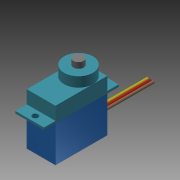
# Autodesk Inventor part: servo-micro tower pro 9g
Saved by Autodesk Inventor 2015 SP2 (Build 190223200, 223)
## iProperties
Created: 2015-05-24
Part Number: servo-micro tower pro 9g
Material: Generic
Document SubType Name: Modeling
Designer: caleb
Density: 1 g/cm^3
Appearance: Default
Author: caleb
Autodesk Inventor part; units mm, degrees
ref_plane "YZ Plane" through (0, 0, 0) normal (1, 0, 0) x (0, 1, 0)
ref_plane "XZ Plane" through (0, 0, 0) normal (0, 1, 0) x (-1, 0, 0)
ref_plane "XY Plane" through (0, 0, 0) normal (0, 0, 1) x (1, 0, 0)
sketch "Sketch1" plane through (0, 0, 0) normal (0, 0, 1) x (1, 0, 0)
  line L0 (-6.35, -16.51) -> (6.35, -16.51)
  line L1 (6.35, -16.51) -> (6.35, 0)
  line L2 (6.35, 6.35) -> (-6.35, 6.35)
  line L3 (-6.35, 6.35) -> (-6.35, 0)
  circle A0 centre (0, 0) radius 6.35
  line L4 (-6.35, 0) -> (-6.35, -16.51)
  line L5 (6.35, 0) -> (6.35, 6.35)
  circle A1 centre (0, 0) radius 2.286
  point P0 (0, 6.35)
  dimension "d0" = 12.7
  dimension "d1" = 22.86
  dimension "d3" = 4.572
  constraints: 12 end point, 5 parallel, 3 tangent, 2 centre point, 2 coincident, 2 perpendicular, 2 point on circle, 1 horizontal, 1 midpoint, 1 vertical alignment
  measures "d0" distance of L0.start L0.end
  measures "d1" distance of L0.end L2.start
  measures "d3" diameter of A1
extrude "Extrusion1" add sketch "Sketch1" against normal blind 16.002 contours L4 A0 L1 L0 | A0 | L3 L2 A0 | A0 L2 L5 | A1
extrude "Extrusion2" add sketch "Sketch1" along normal blind 6.731 separate body contours L4 A0 L1 L0 | A0 | L3 L2 A0 | A0 L2 L5 | A1
sketch "Sketch2" plane through (0, 0, 6.731) normal (0, 0, 1) x (1, 0, 0)
  circle A0 centre (0, 0) radius 6.35 projected
  circle A1 centre (0, 0) radius 2.286 projected
sketch "Sketch3" plane through (0, 0, 0) normal (0, 0, 1) x (1, 0, 0)
  line L0 (-6.35, 6.35) -> (6.35, 6.35)
  line L1 (6.35, 6.35) -> (6.35, 11.43)
  line L2 (6.35, 11.43) -> (-6.35, 11.43)
  line L3 (-6.35, 11.43) -> (-6.35, 6.35)
  line L4 (-6.35, -16.51) -> (6.35, -16.51)
  line L5 (6.35, -16.51) -> (6.35, -21.59)
  line L6 (6.35, -21.59) -> (-6.35, -21.59)
  line L7 (-6.35, -21.59) -> (-6.35, -16.51)
  line L8 (6.35, -16.51) -> (6.35, 6.35) projected
  point P0 (0, 0)
  dimension "d8" = 5.08
  constraints: 16 end point, 4 parallel, 2 coincident, 2 collinear, 2 horizontal, 2 perpendicular
  measures "d8" distance of L4.end L5.end
extrude "Extrusion3" add sketch "Sketch3" along normal blind 0.95 bodies 2
sketch "Sketch4" plane through (0, 0, 0.95) normal (0, 0, 1) x (1, 0, 0)
  line L0 (6.35, 6.35) -> (-6.35, 6.35) projected
  line L1 (6.35, 6.35) -> (6.35, 11.43) projected
  line L2 (6.35, 11.43) -> (-6.35, 11.43) projected
  line L3 (-6.35, 11.43) -> (-6.35, 6.35) projected
  line L4 (-6.35, -16.51) -> (6.35, -16.51) projected
  line L5 (-6.35, -16.51) -> (-6.35, -21.59) projected
  line L6 (-6.35, -21.59) -> (6.35, -21.59) projected
  line L7 (6.35, -21.59) -> (6.35, -16.51) projected
  circle A0 centre (0, 8.89) radius 1.27
  circle A1 centre (0, -19.05) radius 1.27
  point P0 (0, 0)
  point P1 (0, 11.43)
  point P2 (0, -21.59)
  point P3 (6.35, -19.05)
  point P4 (6.35, 8.89)
  dimension "d11" = 2.54
  constraints: 4 midpoint, 2 centre point, 2 horizontal alignment, 2 vertical alignment, 1 equal radius
  measures "d11" diameter of A1
extrude "Extrusion4" cut sketch "Sketch4" against normal through all contours A0 | A1 bodies 2
extrude "Extrusion5" add sketch "Sketch2" along normal blind 4.3434 contours A0 | A1 bodies 2
sketch "Sketch5" plane through (0, 0, 11.0744) normal (0, 0, 1) x (1, 0, 0)
  circle A0 centre (0, 0) radius 2.286 projected
extrude "Extrusion6" add sketch "Sketch5" along normal blind 2.54 separate body
sketch "Sketch6" plane through (-6.35, 6.35, 0) normal (0, 1, 0) x (1, 0, 0)
  line L0 (12.7, 0) -> (0, 0) projected
  line L1 (12.7, 0) -> (12.7, 16.002) projected
  line L2 (0, 16.002) -> (12.7, 16.002) projected
  line L3 (0, 0) -> (0, 16.002) projected
  circle A0 centre (7.5692, 10.8712) radius 0.6096
  circle A1 centre (6.35, 10.8712) radius 0.6096
  circle A2 centre (5.1308, 10.8712) radius 0.6096
  line L4 (6.35, 10.8712) -> (6.35, 11.4808) construction
  line L5 (6.35, 11.4808) -> (6.35, 16.002) construction
  point P0 (6.35, 0)
  dimension "d18" = 1.2192
  dimension "d19" = 4.5212
  constraints: 4 end point, 2 centre point, 2 horizontal alignment, 2 vertical alignment, 1 collinear, 1 midpoint, 1 vertical, 6 other
  measures "d19" distance of L4.end L5.end
extrude "Extrusion7" add sketch "Sketch6" along normal blind 25.4 separate body contours A0
extrude "Extrusion8" add sketch "Sketch6" along normal up to surface (25.4 mm away) separate body contours A1
extrude "Extrusion9" add sketch "Sketch6" along normal up to surface (25.4 mm away) separate body contours A2
body "Solid1"
body "Solid2"
body "Solid3"
body "Solid4"
body "Solid5"
body "Solid6"
